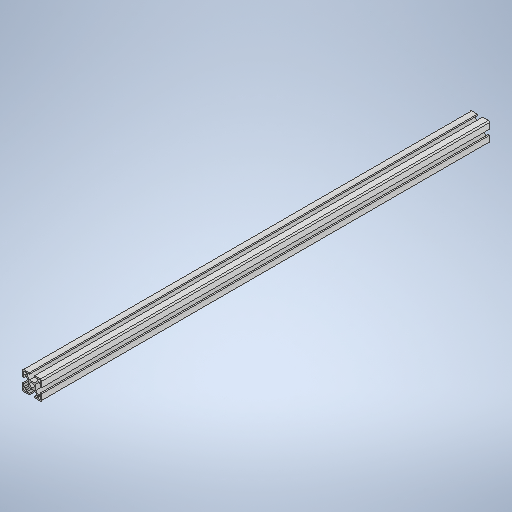
# Autodesk Inventor part: Metal_Profile 70cm
Saved by Autodesk Inventor 2025 (Build 290162000, 162)
## iProperties
Created: 2024-06-13
Part Number: Metal_Profile 70cm
Material: Aluminum 6061-AHC
Document SubType Name: Modeling
Designer: User
Density: 2.7 g/cm^3
Appearance: Default
Author: User
Autodesk Inventor part; units mm, degrees
ref_plane "YZ Plane" through (0, 0, 0) normal (1, 0, 0) x (0, 1, 0)
ref_plane "XZ Plane" through (0, 0, 0) normal (0, 1, 0) x (-1, 0, 0)
ref_plane "XY Plane" through (0, 0, 0) normal (0, 0, 1) x (1, 0, 0)
sketch "Sketch1" plane through (0, 0, 0) normal (0, 0, 1) x (1, 0, 0)
  circle A0 centre (-11.375, 11.375) radius 2.1
  circle A1 centre (-11.375, -11.375) radius 2.1
  line L0 (-15, 4.1) -> (-12.9, 4.1)
  line L1 (-12.9, 4.1) -> (-12.9, 8.28)
  line L2 (-12.9, 8.28) -> (-9.85, 8.28)
  line L3 (-9.85, 8.28) -> (-5.8, 4.23)
  line L4 (-5.8, 4.23) -> (-5.8, -4.23)
  line L5 (-5.8, -4.23) -> (-9.85, -8.28)
  line L6 (-9.85, -8.28) -> (-12.9, -8.28)
  line L7 (-12.9, -8.28) -> (-12.9, -4.1)
  line L8 (-12.9, -4.1) -> (-15, -4.1)
  line L9 (-15, -4.1) -> (-15, -13)
  arc A2 (-15, -13) -> (-13, -15) centre (-13, -13) ccw
  line L10 (-13, -15) -> (-4.1, -15)
  line L11 (-4.1, -15) -> (-4.1, -12.9)
  line L12 (-4.1, -12.9) -> (-8.28, -12.9)
  line L13 (-8.28, -12.9) -> (-8.28, -9.85)
  line L14 (-8.28, -9.85) -> (-3.719, -5.289)
  line L15 (-3.719, -5.289) -> (3.719, -5.289)
  line L16 (3.719, -5.289) -> (8.28, -9.85)
  line L17 (8.28, -9.85) -> (8.28, -12.9)
  line L18 (8.28, -12.9) -> (4.1, -12.9)
  line L19 (4.1, -12.9) -> (4.1, -15)
  line L20 (4.1, -15) -> (13, -15)
  arc A3 (13, -15) -> (15, -13) centre (13, -13) ccw
  line L21 (15, -13) -> (15, -4.1)
  line L22 (15, -4.1) -> (12.9, -4.1)
  line L23 (12.9, -4.1) -> (12.9, -8.28)
  line L24 (12.9, -8.28) -> (9.85, -8.28)
  line L25 (9.85, -8.28) -> (5.8, -4.23)
  line L26 (5.8, -4.23) -> (5.8, 4.23)
  line L27 (5.8, 4.23) -> (9.85, 8.28)
  line L28 (9.85, 8.28) -> (12.9, 8.28)
  line L29 (12.9, 8.28) -> (12.9, 4.1)
  line L30 (12.9, 4.1) -> (15, 4.1)
  line L31 (15, 4.1) -> (15, 13)
  arc A4 (15, 13) -> (13, 15) centre (13, 13) ccw
  line L32 (13, 15) -> (4.1, 15)
  line L33 (4.1, 15) -> (4.1, 12.9)
  line L34 (4.1, 12.9) -> (8.28, 12.9)
  line L35 (8.28, 12.9) -> (8.28, 9.85)
  line L36 (8.28, 9.85) -> (3.719, 5.289)
  line L37 (3.719, 5.289) -> (-3.719, 5.289)
  line L38 (-3.719, 5.289) -> (-8.28, 9.85)
  line L39 (-8.28, 9.85) -> (-8.28, 12.9)
  line L40 (-8.28, 12.9) -> (-4.1, 12.9)
  line L41 (-4.1, 12.9) -> (-4.1, 15)
  line L42 (-4.1, 15) -> (-13, 15)
  arc A5 (-13, 15) -> (-15, 13) centre (-13, 13) ccw
  line L43 (-15, 13) -> (-15, 4.1)
  circle A6 centre (0, 0) radius 3.4
  circle A7 centre (11.375, 11.375) radius 2.1
  circle A8 centre (11.375, -11.375) radius 2.1
  constraints: 88 end point, 9 centre point, 8 point on circle, 2 coincident
extrude "Extrusion1" add sketch "Sketch1" against normal blind 700
body "Solid1"
